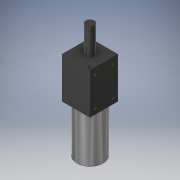
# Autodesk Inventor part: micro cim
Saved by Autodesk Inventor 2017 SP1 (Build 210196100, 196)
## iProperties
Created: 2018-01-26
Part Number: micro cim
Material: Generic
Document SubType Name: Modeling
Designer: Ben
Density: 1 g/cm^3
Appearance: Smooth - Black
Author: Ben
Autodesk Inventor part; units mm, degrees
ref_plane "YZ Plane" through (0, 0, 0) normal (1, 0, 0) x (0, 1, 0)
ref_plane "XZ Plane" through (0, 0, 0) normal (0, 1, 0) x (-1, 0, 0)
ref_plane "XY Plane" through (0, 0, 0) normal (0, 0, 1) x (1, 0, 0)
sketch "Sketch1" plane through (0, 0, 0) normal (0, 1, 0) x (-1, 0, 0)
  line L0 (-20.955, 20.955) -> (20.955, 20.955)
  line L1 (20.955, 20.955) -> (20.955, -20.955)
  line L2 (20.955, -20.955) -> (-20.955, -20.955)
  line L3 (-20.955, -20.955) -> (-20.955, 20.955)
  line L4 (-20.955, 20.955) -> (20.955, -20.955) construction
  line L5 (20.955, 20.955) -> (-20.955, -20.955) construction
  circle A0 centre (17.4625, -17.4625) radius 2.54
  circle A1 centre (-17.4625, 17.4625) radius 2.54
  line L6 (17.4625, -17.4625) -> (17.4625, 17.4625) construction
  line L7 (-17.4625, 17.4625) -> (-17.4625, -17.4625) construction
  line L8 (0, 20.955) -> (0, -20.955) construction
  point P0 (0, 0)
  dimension "d0" = 41.91
  dimension "d1" = 34.925
  dimension "d2" = 5.08
  constraints: 18 end point, 4 midpoint, 4 point on line, 3 parallel, 2 centre point, 2 equal length, 1 equal radius, 1 horizontal, 1 perpendicular, 1 vertical
  measures "d0" distance of L1.end L2.end
  measures "d1" distance of L6.start L6.end
  measures "d2" diameter of A0
extrude "Extrusion1" add sketch "Sketch1" along normal blind 62.23
sketch "Sketch2" plane through (0, 0, 0) normal (0, -1, 0) x (1, 0, 0)
  circle A0 centre (0, 0) radius 19.812
  dimension "d5" = 39.624
  constraints: 1 centre point, 1 coincident
  measures "d5" diameter of A0
extrude "Extrusion2" add sketch "Sketch2" along normal blind 71.12
sketch "Sketch3" plane through (0, -71.12, 0) normal (0, -1, 0) x (1, 0, 0)
  circle A0 centre (0, 0) radius 6.35
  dimension "d8" = 12.7
  constraints: 1 centre point, 1 coincident
  measures "d8" diameter of A0
extrude "Extrusion3" add sketch "Sketch3" along normal blind 1.524
sketch "Sketch4" plane through (0, 62.23, 0) normal (0, 1, 0) x (1, 0, 0)
  circle A0 centre (0, 0) radius 6.35
  dimension "d11" = 12.7
  constraints: 1 centre point, 1 coincident
  measures "d11" diameter of A0
extrude "Extrusion4" add sketch "Sketch4" along normal blind 40.64
sketch "Sketch5" plane through (20.955, 0, 20.955) normal (1, 0, 0) x (0, 0, -1)
  line L0 (8.255, 52.07) -> (33.655, 52.07) construction
  line L1 (33.655, 52.07) -> (33.655, 7.62) construction
  line L2 (33.655, 7.62) -> (8.255, 7.62) construction
  line L3 (8.255, 7.62) -> (8.255, 52.07) construction
  line L4 (20.955, 0) -> (20.955, 7.62) construction
  line L5 (0, 62.23) -> (41.91, 62.23) construction
  circle A0 centre (8.255, 52.07) radius 1.905
  circle A1 centre (33.655, 52.07) radius 1.905
  circle A2 centre (33.655, 7.62) radius 1.905
  circle A3 centre (8.255, 7.62) radius 1.905
  dimension "d14" = 25.4
  dimension "d15" = 44.45
  dimension "d16" = 10.16
  dimension "d17" = 3.81
  constraints: 10 end point, 4 centre point, 4 coincident, 3 equal radius, 2 parallel, 1 horizontal, 1 midpoint, 1 perpendicular, 1 vertical
  measures "d14" distance of L0.start L0.end
  measures "d15" distance of L0.end L1.end
  measures "d16" distance between parallel lines of L0 L5
  measures "d17" diameter of A0
extrude "Extrusion5" cut sketch "Sketch5" against normal through all
body "Solid1"
